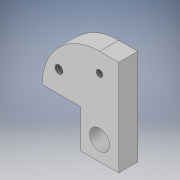
# Autodesk Inventor part: Shooter_Stop
Saved by Autodesk Inventor 2019 (Build 230136000, 136)
## iProperties
Created: 2019-04-04
Part Number: Shooter_Stop
Material: Generic
Document SubType Name: Modeling
Designer: Delta
Density: 1 g/cm^3
Appearance: Default
Author: Delta
Autodesk Inventor part; units mm, degrees
ref_plane "YZ Plane" through (0, 0, 0) normal (1, 0, 0) x (0, 1, 0)
ref_plane "XZ Plane" through (0, 0, 0) normal (0, 1, 0) x (-1, 0, 0)
ref_plane "XY Plane" through (0, 0, 0) normal (0, 0, 1) x (1, 0, 0)
sketch "Sketch1" plane through (0, 0, 0) normal (0, 0, 1) x (1, 0, 0)
  line L0 (0, 0) -> (12.7, 0)
  line L1 (12.7, 0) -> (12.7, 31.75)
  line L2 (12.7, 31.75) -> (0, 31.75)
  line L3 (0, 12.7) -> (0, 0)
  line L4 (12.7, 31.75) -> (-12.7, 31.75)
  line L5 (-12.7, 31.75) -> (-12.7, 12.7)
  line L6 (-12.7, 12.7) -> (0, 12.7)
  line L7 (12.7, 12.7) -> (12.7, 31.75)
  dimension "d1" = 31.75
  dimension "d2" = 25.4
  dimension "d3" = 19.05
  dimension "d4" = 12.7
  dimension "d5" = 12.7
  constraints: 16 end point, 4 parallel, 2 horizontal, 2 perpendicular
  measures "d1" distance of L1.end L0.end
  measures "d2" distance of L7.start L5.end
  measures "d3" distance of L5.end L4.end
  measures "d4" distance between parallel lines of L3 L5
  measures "d5" distance between parallel lines of L3 L1
extrude "Extrusion1" add sketch "Sketch1" along normal blind 6.35
fillet "Fillet1" radius 19.05 1 edges at (-12.7, 31.75, 3.175)
sketch "Sketch2" plane through (0, 0, 6.35) normal (0, 0, 1) x (1, 0, 0)
  line L0 (12.7, 0) -> (12.7, 31.75) projected
  line L1 (0, 0) -> (12.7, 0) projected
  point P0 (6.35, 6.35)
  dimension "d11" = 6.35
  dimension "d12" = 6.35
  measures "d11" distance from line of L0 point (6.35, 6.35)
  measures "d12" distance from line of L1 point (6.35, 6.35)
hole "Hole1" at (6.35, 6.35, 6.35) direction (0, 0, -1) diameter 6.604 end through all
sketch "Sketch3" plane through (0, 0, 6.35) normal (0, 0, 1) x (1, 0, 0)
  line L0 (12.7, 0) -> (12.7, 31.75) projected
  line L1 (12.7, 31.75) -> (6.35, 31.75) projected
  point P0 (0, 0)
  point P1 (6.35, 25.4)
  dimension "d20" = 6.35
  dimension "d21" = 6.35
  measures "d20" distance from line of point (6.35, 25.4) L0
  measures "d21" distance from line of point (6.35, 25.4) L1
hole "Hole2" at (6.35, 25.4, 6.35) direction (0, 0, -1) diameter 2.159 end through all
sketch "Sketch4" plane through (0, 0, 6.35) normal (0, 0, 1) x (1, 0, 0)
  circle A0 centre (6.35, 6.35) radius 3.302 projected
  circle A1 centre (6.35, 6.35) radius 19.05
  line L0 (-7.1204, 19.8204) -> (6.35, 6.35)
  line L1 (12.7, 0) -> (12.7, 31.75) projected
  point P0 (0, 0)
  dimension "d29" = 38.1
  dimension "d30" = 45
  constraints: 2 end point, 1 coincident, 3 other
  measures "d30" angle of L1 L0
hole "Hole3" at (-7.1204, 19.8204, 6.35) direction (0, 0, -1) diameter 2.6416 end through all thread size "6-32 UNC" class "2B" standard "ANSI Unified Screw Threads"
equation "\"d12\" = d11"
equation "\"d21\" = d20"
body "Solid1"
